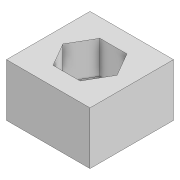
# Autodesk Inventor part: M4 net well test
Saved by Autodesk Inventor 2020 (Build 240168000, 168)
## iProperties
Created: 2020-03-04
Part Number: M4 net well test
Material: Generic
Document SubType Name: Modeling
Designer: ball
Density: 1 g/cm^3
Appearance: Default
Author: ball
Autodesk Inventor part; units mm, degrees
ref_plane "YZ Plane" through (0, 0, 0) normal (1, 0, 0) x (0, 1, 0)
ref_plane "XZ Plane" through (0, 0, 0) normal (0, 1, 0) x (-1, 0, 0)
ref_plane "XY Plane" through (0, 0, 0) normal (0, 0, 1) x (1, 0, 0)
sketch "Sketch1" plane through (0, 0, 0) normal (0, 1, 0) x (-1, 0, 0)
  line L0 (6.35, 6.35) -> (-6.35, 6.35)
  line L1 (-6.35, 6.35) -> (-6.35, -6.35)
  line L2 (-6.35, -6.35) -> (6.35, -6.35)
  line L3 (6.35, -6.35) -> (6.35, 6.35)
  line L4 (6.35, 6.35) -> (-6.35, -6.35) construction
  line L5 (-6.35, 6.35) -> (6.35, -6.35) construction
  circle A0 centre (0, 0) radius 2.2
  dimension "d0" = 12.7
  dimension "d1" = 12.7
  dimension "d2" = 4.4
  constraints: 12 end point, 2 midpoint, 2 parallel, 1 centre point, 1 coincident, 1 horizontal, 1 perpendicular
  measures "d0" distance of L2.end L1.end
  measures "d1" distance of L1.end L0.end
  measures "d2" diameter of A0
extrude "Extrusion1" add sketch "Sketch1" along normal blind 8
sketch "Sketch2" plane through (0, 8, 0) normal (0, 1, 0) x (1, 0, 0)
  circle A0 centre (0, 0) radius 4.115 construction
  line L0 (4.115, 0) -> (2.0575, -3.5637)
  line L1 (2.0575, -3.5637) -> (-2.0575, -3.5637)
  line L2 (-2.0575, -3.5637) -> (-4.115, 0)
  line L3 (-4.115, 0) -> (-2.0575, 3.5637)
  line L4 (-2.0575, 3.5637) -> (2.0575, 3.5637)
  line L5 (2.0575, 3.5637) -> (4.115, 0)
  dimension "d5" = 8.23
  constraints: 12 end point, 2 coincident, 1 horizontal alignment, 15 other
extrude "Extrusion2" cut sketch "Sketch2" against normal blind 5
body "Solid1"
